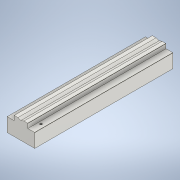
# Autodesk Inventor part: Base soporte tubos
Saved by Autodesk Inventor 2021 (Build 250183000, 183)
## iProperties
Created: 2021-04-30
Part Number: Base soporte tubos
Material: Steel AISI 1045 HV HR
Document SubType Name: Modeling
Designer: Nelson
Density: 7.85 g/cm^3
Appearance: Steel
Mass: 181117 g
Surface Area: 7176.3 cm^2
Volume: 23072.2 cm^3
Author: Nelson
Autodesk Inventor part; units mm, degrees
ref_plane "YZ Plane" through (0, 0, 0) normal (1, 0, 0) x (0, 1, 0)
ref_plane "XZ Plane" through (0, 0, 0) normal (0, 1, 0) x (-1, 0, 0)
ref_plane "XY Plane" through (0, 0, 0) normal (0, 0, 1) x (1, 0, 0)
sketch "Sketch1" plane through (0, 0, 0) normal (0, 0, 1) x (1, 0, 0)
  line L0 (-50, 100) -> (-50, 132.5)
  line L1 (50, 100) -> (50, 132.5)
  line L2 (-21.6183, 132.5) -> (0, 125)
  line L3 (0, 125) -> (21.6183, 132.5)
  line L4 (-100, 100) -> (-50, 100)
  line L5 (50, 100) -> (100, 100)
  line L6 (0, 125) -> (0, 131.5) construction
  line L7 (-21.6183, 132.5) -> (-50, 132.5)
  line L8 (21.6183, 132.5) -> (50, 132.5)
  line L9 (-100, 100) -> (-100, 0)
  line L10 (100, 0) -> (100, 100)
  line L11 (-100, 0) -> (0, 0)
  line L12 (0, 0) -> (100, 0)
  dimension "d90" = 32.5
  dimension "d91" = 50
  dimension "d92" = 50
  dimension "d105" = 25
  dimension "d108" = 100
  dimension "d110" = 50
  constraints: 26 end point, 5 equal length, 5 horizontal, 5 vertical, 1 collinear
  measures "d90" distance of L0.start L0.end
  measures "d91" distance from line of L11.end L0
  measures "d92" distance from line of L11.end L1
  measures "d105" distance from line of L4 L2.end
  measures "d108" distance of L4.start L9.end
  measures "d110" distance of L4.start L0.start
extrude "Extrusion1" add sketch "Sketch1" against normal blind 1000
sketch "Sketch4" plane through (-100, 100, 0) normal (0, 1, 0) x (1, 0, 0)
  line L0 (0, 0) -> (0, 1000) projected
  line L1 (50, 0) -> (0, 0) projected
  line L2 (200, 0) -> (200, 1000) projected
  line L3 (200, 0) -> (150, 0) projected
  point P0 (100, 0)
  point P1 (30, 75)
  point P2 (170, 75)
  dimension "d63" = 30
  dimension "d64" = 75
  dimension "d65" = 30
  dimension "d109" = 75
  measures "d63" distance from line of L0 point (30, 75)
  measures "d64" distance from line of L3 point (170, 75)
  measures "d65" distance from line of L2 point (170, 75)
  measures "d109" distance from line of L1 point (30, 75)
hole "Hole2" at (-70, 100, -75) at (70, 100, -75) direction (0, -1, 0) diameter 15.875 depth 20 tip angle 137
thread "Thread1" size "5/8-11 UNC" class "2B" standard "ANSI Unified Screw Threads" full length
thread "Thread2" size "5/8-11 UNC" class "2B" standard "ANSI Unified Screw Threads" length 70
chamfer "Chamfer1" distance 1 angle 45 4 edges at (-50, 132.5, -500) (-100, 100, -500) (50, 132.5, -500) (100, 100, -500)
sketch "Sketch6" plane through (-100, 0, 0) normal (0, -1, 0) x (1, 0, 0)
  line L0 (200, 0) -> (200, -1000) projected
  line L1 (190, -60) -> (190, -115.207) construction
  line L2 (190, -60) -> (167.102, -60) construction
  line L3 (167.102, -60) -> (167.102, -115.207) construction
  line L4 (100, 0) -> (100, -1000) construction
  line L5 (10, -60) -> (10, -115.207) construction
  line L6 (10, -60) -> (32.898, -60) construction
  line L7 (32.898, -60) -> (32.898, -115.207) construction
  line L8 (200, -500) -> (0, -500) construction
  line L9 (0, 0) -> (0, -1000) construction
  line L10 (190, -940) -> (190, -884.793) construction
  line L11 (190, -940) -> (167.102, -940) construction
  line L12 (167.102, -940) -> (167.102, -884.793) construction
  line L13 (10, -940) -> (10, -884.793) construction
  line L14 (32.898, -940) -> (32.898, -884.793) construction
  line L15 (10, -940) -> (32.898, -940) construction
  line L16 (0, 0) -> (200, 0) construction
  dimension "d111" = 10
  dimension "d112" = 55.207
  dimension "d113" = 22.898
  dimension "d115" = 60
  constraints: 26 end point, 21 symmetric about line, 12 coincident, 2 midpoint, 1 horizontal, 1 parallel, 1 perpendicular, 1 vertical
  measures "d111" distance from line of L0 L1.start
  measures "d112" distance of L1.start L1.end
  measures "d113" distance of L1.start L2.end
  measures "d115" distance from line of L1.start L16
hole "Hole3" at (90, 0, -60) at (90, 0, -115.207) at (67.102, 0, -60) at (67.102, 0, -115.207) at (-90, 0, -60) at (-90, 0, -115.207) at (-67.102, 0, -60) at (-67.102, 0, -115.207) at (90, 0, -940) at (90, 0, -884.793) at (67.102, 0, -940) at (67.102, 0, -884.793) at (-67.102, 0, -940) at (-67.102, 0, -884.793) at (-90, 0, -940) at (-90, 0, -884.793) direction (0, 1, 0) diameter 4.917 depth 17.1 tip angle 137 thread size "M6x1" class "6H" standard "ISO Metric profile"
equation "\"d92\" = d91"
equation "\"d64\" = d62"
equation "\"d65\" = d63"
equation "\"d36\" = d34"
equation "\"d34\" = 75"
equation "\"d62\" = 75"
body "Solid1"
